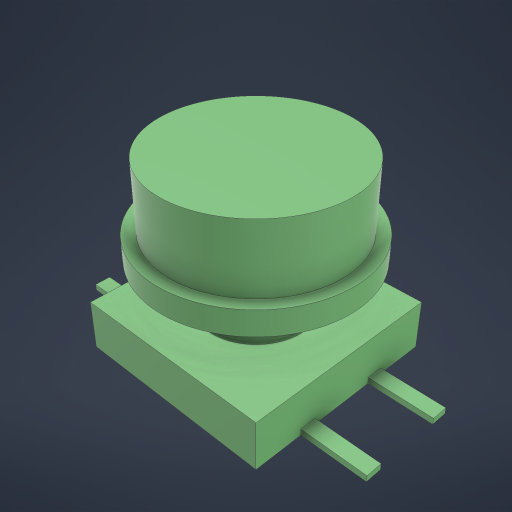
# Autodesk Inventor part: Button
Saved by Autodesk Inventor 2023 (Build 270158030, 158C)
## iProperties
Created: 2022-04-28
Part Number: Button
Material: Generic
Document SubType Name: Modeling
Designer: Simon
Density: 1 g/cm^3
Appearance: Default
Author: Simon
Autodesk Inventor part; units mm, degrees
ref_plane "YZ Plane" through (0, 0, 0) normal (1, 0, 0) x (0, 1, 0)
ref_plane "XZ Plane" through (0, 0, 0) normal (0, 1, 0) x (-1, 0, 0)
ref_plane "XY Plane" through (0, 0, 0) normal (0, 0, 1) x (1, 0, 0)
sketch "Sketch3" plane through (0, 0, 0) normal (0, 1, 0) x (-1, 0, 0)
  line L0 (6, 6) -> (-6, 6)
  line L1 (-6, 6) -> (-6, -6)
  line L2 (-6, -6) -> (6, -6)
  line L3 (6, -6) -> (6, 6)
  line L4 (6, 6) -> (-6, -6) construction
  line L5 (-6, 6) -> (6, -6) construction
  point P0 (0, 0)
  dimension "d7" = 12
  dimension "d8" = 12
  constraints: 12 end point, 2 midpoint, 2 parallel, 1 horizontal, 1 perpendicular
  measures "d7" distance of L2.end L1.end
  measures "d8" distance of L1.end L0.end
extrude "Extrusion3" add sketch "Sketch3" along normal blind 3
sketch "Sketch4" plane through (0, 3, 0) normal (0, 1, 0) x (1, 0, 0)
  circle A0 centre (0, 0) radius 3.3
  dimension "d11" = 6.6
  constraints: 1 centre point, 1 coincident
  measures "d11" diameter of A0
extrude "Extrusion4" add sketch "Sketch4" along normal blind 3.2
sketch "Sketch5" plane through (0, 6.2, 0) normal (0, 1, 0) x (1, 0, 0)
  circle A0 centre (0, 0) radius 6.5
  dimension "d14" = 13
  constraints: 1 centre point, 1 coincident
  measures "d14" diameter of A0
extrude "Extrusion5" add sketch "Sketch5" along normal blind 1.5
sketch "Sketch6" plane through (0, 7.7, 0) normal (0, 1, 0) x (1, 0, 0)
  circle A0 centre (0, 0) radius 5.75
  dimension "d17" = 11.5
  constraints: 1 centre point, 1 coincident
  measures "d17" diameter of A0
extrude "Extrusion6" add sketch "Sketch6" along normal blind 4.1
sketch "Sketch7" plane through (-6, 0, -6) normal (-1, 0, 0) x (0, 0, 1)
  line L0 (3, -0.4) -> (9, -0.4)
  line L1 (9, -0.4) -> (9, 0.4)
  line L2 (9, 0.4) -> (3, 0.4)
  line L3 (3, 0.4) -> (3, -0.4)
  line L4 (3, -0.4) -> (9, 0.4) construction
  line L5 (9, -0.4) -> (3, 0.4) construction
  line L6 (4, -0.4) -> (8, -0.4)
  line L7 (8, -0.4) -> (8, 0.4)
  line L8 (8, 0.4) -> (4, 0.4)
  line L9 (4, 0.4) -> (4, -0.4)
  line L10 (4, -0.4) -> (8, 0.4) construction
  line L11 (8, -0.4) -> (4, 0.4) construction
  line L12 (0, 0) -> (12, 0) projected
  point P0 (6, 0)
  point P1 (8, 0)
  point P2 (9, 0)
  point P3 (3, 0)
  point P4 (4, 0)
  dimension "d20" = 6
  dimension "d21" = 0.8
  dimension "d22" = 4
  constraints: 24 end point, 4 midpoint, 4 parallel, 2 horizontal, 2 perpendicular, 1 point on line
  measures "d20" distance of L2.end L1.end
  measures "d21" distance of L1.end L0.end
  measures "d22" distance of L8.end L7.end
extrude "Extrusion7" add sketch "Sketch7" along normal blind 4 contours L3 L2 L9 L12 | L7 L2 L1 L12
mirror "Mirror1" about plane through (0, 0, 0) normal (1, 0, 0) of "Extrusion7"
body "Solid2"
